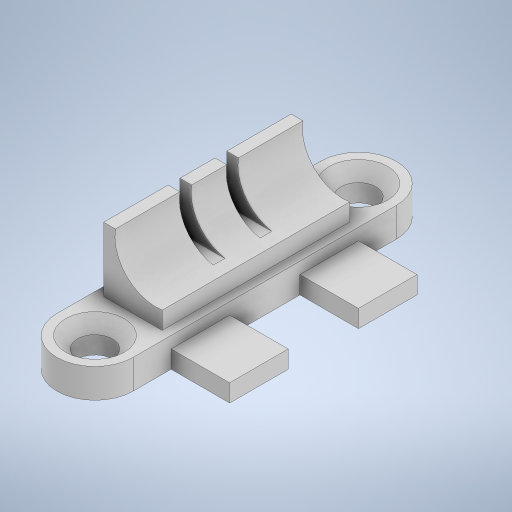
# Autodesk Inventor part: string_holderWPNB
Saved by Autodesk Inventor 2024 (Build 280153000, 153)
## iProperties
Created: 2025-10-10
Part Number: string_holderWPNB
Material: Generic
Document SubType Name: Modeling
Designer: albah
Density: 1 g/cm^3
Appearance: Default
Author: albah
Autodesk Inventor part; units mm, degrees
ref_plane "YZ Plane" through (0, 0, 0) normal (1, 0, 0) x (0, 1, 0)
ref_plane "XZ Plane" through (0, 0, 0) normal (0, 1, 0) x (-1, 0, 0)
ref_plane "XY Plane" through (0, 0, 0) normal (0, 0, 1) x (1, 0, 0)
sketch "Sketch1" plane through (0, 0, 0) normal (0, 1, 0) x (-1, 0, 0)
  line L0 (-6.5, 22.5) -> (-6.5, -22.5)
  line L1 (-6.5, -22.5) -> (6.5, -22.5)
  line L2 (6.5, -22.5) -> (6.5, 22.5)
  line L3 (6.5, 22.5) -> (-6.5, 22.5)
  line L4 (-6.5, 22.5) -> (6.5, -22.5) construction
  line L5 (-6.5, -22.5) -> (6.5, 22.5) construction
  circle A0 centre (0, -22.5) radius 3
  circle A1 centre (0, -22.5) radius 6.5
  circle A2 centre (0, 22.5) radius 3
  circle A3 centre (0, 22.5) radius 6.5
  line L6 (-5, 16) -> (-5, -16)
  line L7 (-5, -16) -> (5, -16)
  line L8 (5, -16) -> (5, 16)
  line L9 (5, 16) -> (-5, 16)
  line L10 (-5, 16) -> (5, -16) construction
  line L11 (-5, -16) -> (5, 16) construction
  line L12 (-6.5, -16) -> (-6.5, -6)
  line L13 (-6.5, -6) -> (-16.5, -6)
  line L14 (-16.5, -6) -> (-16.5, -16)
  line L15 (-16.5, -16) -> (-6.5, -16)
  line L16 (-6.5, 16) -> (-6.5, 6)
  line L17 (-6.5, 6) -> (-16.5, 6)
  line L18 (-16.5, 6) -> (-16.5, 16)
  line L19 (-16.5, 16) -> (-6.5, 16)
  point P0 (0, 0)
  dimension "d0" = 45
  dimension "d1" = 13
  dimension "d2" = 6
  dimension "d3" = 6
  dimension "d4" = 10
  dimension "d5" = 10
  dimension "d6" = 10
  dimension "d7" = 10
  dimension "d8" = 10
  constraints: 40 end point, 8 parallel, 6 midpoint, 5 point on line, 4 perpendicular, 3 centre point, 2 coincident, 2 horizontal, 2 vertical, 1 tangent, 3 other
  measures "d0" distance of L0.start L0.end
  measures "d1" distance of L1.end L0.end
  measures "d2" diameter of A0
  measures "d3" diameter of A2
  measures "d4" distance of L7.end L6.end
  measures "d5" distance of L12.start L12.end
  measures "d6" distance of L13.end L12.end
  measures "d7" distance of L16.start L16.end
  measures "d8" distance of L16.end L17.end
extrude "Extrusion1" add sketch "Sketch1" along normal blind 5 contours A3 L9 L6 L7 A1 L0 | A3 L3 A2 | L3 A2 A3 | L2 A1 L7 L8 L9 A3 | A1 L1 A0 | L1 A0 A1
extrude "Extrusion2" add sketch "Sketch1" along normal blind 3 contours L0 L17 L18 L19 | L0 L15 L14 L13
extrude "Extrusion3" add sketch "Sketch1" along normal blind 16 contours L9 L8 L7 L6
sketch "Sketch2" plane through (-5, 5, 16) normal (0, 0, 1) x (1, 0, 0)
  line L0 (10, 11) -> (0, 11) projected
  line L1 (0, 11) -> (2, 11)
  line L2 (10, 0) -> (10, 11) projected
  line L3 (11.5, 0) -> (-1.5, 0) projected
  line L4 (0, 0) -> (0, 11) projected
  arc A0 (2, 11) -> (10, 3) centre (8.8459, 9.8459) ccw
  point P0 (5, -5)
  point P1 (3, 6.101)
  dimension "d15" = 2
  dimension "d16" = 3
  dimension "d17" = 5
  dimension "d18" = 3
  constraints: 3 point on circle, 2 end point, 2 point on line, 1 centre point
  measures "d15" distance of L0.end L1.end
  measures "d16" distance from line of L3 A0.end
  measures "d17" distance of L1.end point (3, 6.101)
  measures "d18" distance from line of L4 point (3, 6.101)
extrude "Extrusion4" cut sketch "Sketch2" against normal through all contours L2 A0 L0
sketch "Sketch3" plane through (-5, 5, 16) normal (-1, 0, 0) x (0, 0, 1)
  line L0 (0, 11) -> (-32, 11) projected
  line L1 (-32, 11) -> (0, 11) projected
  line L2 (0, 0) -> (0, 11) projected
  line L3 (-38.5, 0) -> (6.5, 0) projected
  line L4 (-19, 11) -> (-19, 3)
  line L5 (-19, 3) -> (-32, 3)
  line L6 (-13, 11) -> (-13, 3)
  line L7 (-13, 3) -> (0, 3)
  line L8 (-32, 3) -> (-19, 3)
  line L9 (-19, 3) -> (-19, 11)
  line L10 (-19, 11) -> (-32, 11)
  line L11 (-32, 11) -> (-32, 3)
  line L12 (-13, 3) -> (0, 3)
  line L13 (0, 3) -> (0, 11)
  line L14 (0, 11) -> (-13, 11)
  line L15 (-13, 11) -> (-13, 3)
  line L16 (-21, 3) -> (-21, 11)
  line L17 (-11, 11) -> (-11, 3)
  point P0 (-16, -5)
  point P1 (-16, 11)
  point P2 (-16, 11)
  point P3 (-16, 11)
  point P4 (-11, 3)
  dimension "d21" = 3
  dimension "d22" = 3
  dimension "d23" = 3
  dimension "d24" = 3
  dimension "d25" = 32
  dimension "d26" = 2
  dimension "d27" = 2
  constraints: 28 end point, 7 point on line, 6 perpendicular, 5 equal length, 3 midpoint, 2 vertical, 1 horizontal
  measures "d21" distance of point (-16, 11) L4.start
  measures "d22" distance of point (-16, 11) L6.start
  measures "d23" distance from line of L3 L7.end
  measures "d24" distance from line of L3 L5.end
  measures "d25" distance from line of L5.end L2
  measures "d26" distance between parallel lines of L4 L16
  measures "d27" distance between parallel lines of L17 L6
extrude "Extrusion5" cut sketch "Sketch3" against normal blind 10 contours L4 L5 L16 L0 | L17 L7 L6 L0
chamfer "Chamfer1" distance 2 angle 45 2 edges at (3, 5, -22.5) (3, 5, 22.5)
body "Solid1"
